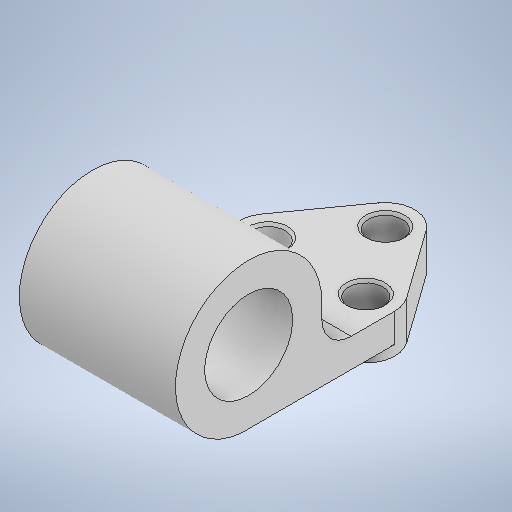
# Autodesk Inventor part: num1
Saved by Autodesk Inventor 2025 (Build 290162000, 162)
## iProperties
Created: 2025-04-26
Part Number: num1
Material: Všeobecné
Document SubType Name: Modeling
Designer: jakub
Density: 1 g/cm^3
Appearance: Výchozí
Author: jakub
Autodesk Inventor part; units mm, degrees
ref_plane "XZ Plane" through (0, 0, 0) normal (0, 1, 0) x (-1, 0, 0)
ref_plane "XY Plane" through (0, 0, 0) normal (0, 0, 1) x (1, 0, 0)
sketch "Sketch1" plane through (0, 0, 0) normal (0, 1, 0) x (-1, 0, 0)
  circle A0 centre (0, 0) radius 7
  circle A1 centre (-40, 0) radius 7
  circle A2 centre (-20, -28) radius 7
  arc A3 (9.7648, -6.9749) -> (0, 12) centre (0, 0) ccw
  arc A4 (-40, 12) -> (-49.7648, -6.9749) centre (-40, 0) ccw
  arc A5 (-29.7648, -34.9749) -> (-10.2352, -34.9749) centre (-20, -28) ccw
  line L0 (0, 12) -> (-40, 12)
  line L1 (-49.7648, -6.9749) -> (-29.7648, -34.9749)
  arc A6 (9.7648, -6.9749) -> (0, 12) centre (0, 0) ccw
  line L2 (9.7648, -6.9749) -> (-10.2352, -34.9749)
  constraints: 8 point on circle, 7 centre point, 6 end point, 4 coincident, 3 tangent, 1 horizontal
extrude "Extrusion1" add sketch "Sketch1" along normal blind 16
ref_plane "Work Plane1" through (20, 0, 0) normal (1, 0, 0) x (0, 1, 0)
sketch "Sketch2" plane through (20, 0, 0) normal (1, 0, 0) x (0, 1, 0)
  line L0 (16, -40) -> (16, -34.9749) projected
  arc A0 (34, 30) -> (4.186, 63.3352) centre (34, 60) ccw
  line L1 (4.186, 63.3352) -> (4.186, 12)
  line L2 (0, 12) -> (16, 12) projected
  line L3 (16, -6.9749) -> (16, 12) projected
  line L4 (16, 12) -> (16, 18)
  line L5 (0, 12) -> (4, 12)
  line L6 (34, 30) -> (28, 30)
  circle A1 centre (34, 60) radius 18
  arc A2 (28, 30) -> (16, 18) centre (28, 18) ccw
  point P0 (0, 0)
  dimension "d36" = 12
  constraints: 8 end point, 4 point on circle, 3 centre point, 2 point on line, 2 vertical, 1 coincident, 1 collinear, 1 horizontal, 1 tangent
  measures "d36" radius of A2
extrude "Extrusion2" add sketch "Sketch2" along normal mid plane 64
sketch "Sketch3" plane through (0, 4.186, 12) normal (0, 0, -1) x (-1, 0, 0)
  line L0 (12, 11.814) -> (0, 11.814) projected
  line L1 (-40, 0) -> (0, 0) projected
  line L2 (12, 11.814) -> (0, 11.814)
  line L3 (0, 11.814) -> (0, 0)
  line L4 (0, 0) -> (12, 0)
  line L5 (12, 0) -> (12, 11.814)
  point P0 (0, -4.186)
  point P1 (0, 11.814)
  constraints: 8 end point, 2 parallel, 1 horizontal, 1 perpendicular
extrude "Extrusion3" add sketch "Sketch3" along normal blind 11.75
sketch "Sketch4" plane through (0, 16, 0) normal (0, 1, 0) x (1, 0, 0)
  point P0 (0, 0)
hole "Hole1" at (0, 16, 0) direction (0, -1, 0) diameter 14 depth 29.1
chamfer "Chamfer1" distance 2 angle 45 2 edges at (-12, 16, 60) (52, 16, 60)
chamfer "Chamfer2" distance 1 angle 45 9 edges at (47, 16, 0) (-4.8606, 16, 5.0374) (-6.9989, 16, 0.125) (4.9497, 16, -4.9497) (27, 16, -28) (47, 0, 0) (27, 0, -28) (-4.9497, 0, 4.9497) (4.9497, 0, -4.9497)
mirror "Mirror3" about plane through (20, 0, 0) normal (1, 0, 0) of "Extrusion2", "Extrusion1", "Chamfer2", "Extrusion3", "Hole1"
body "Solid1"
